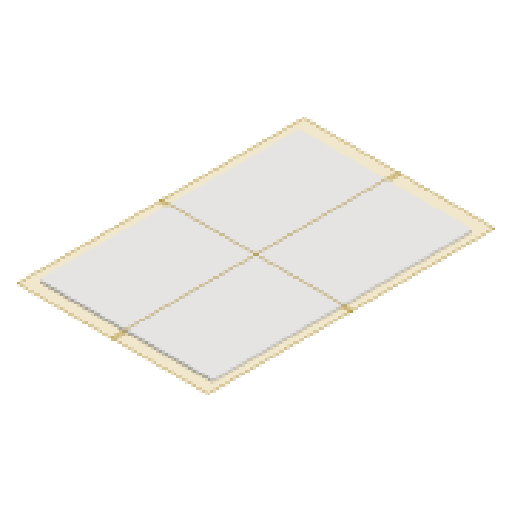
# Autodesk Inventor part: platform
Saved by Autodesk Inventor 2023.2 (Build 272271030, 271C)
## iProperties
Created: 2024-10-30
Part Number: platform
Material: Типовые
Document SubType Name: Modeling
Designer: I9232
Density: 1 g/cm^3
Appearance: По умолчанию
Author: I9232
Autodesk Inventor part; units mm, degrees
sketch "Эскиз1" plane through (0, 0, 0) normal (0, 1, 0) x (-1, 0, 0)
  line L0 (200, 300) -> (-200, 300)
  line L1 (-200, 300) -> (-200, -300)
  line L2 (-200, -300) -> (200, -300)
  line L3 (200, -300) -> (200, 300)
  line L4 (200, 300) -> (-200, -300) construction
  line L5 (-200, 300) -> (200, -300) construction
  point P0 (0, 0)
  dimension "d0" = 600
  dimension "d1" = 400
  constraints: 12 end point, 2 midpoint, 2 parallel, 1 horizontal, 1 perpendicular
  measures "d0" distance of L0.end L1.end
  measures "d1" distance of L1.end L2.end
extrude "Выдавливание1" add sketch "Эскиз1" along normal mid plane 6
fillet "Сопряжение1" radius 4 4 edges at (-200, 0, -300) (200, 0, -300) (200, 0, 300) (-200, 0, 300)
